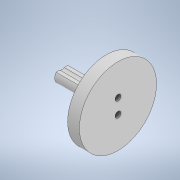
# Autodesk Inventor part: engine_gear_connector
Saved by Autodesk Inventor 2020.1 (Build 241239000, 239)
## iProperties
Created: 2022-03-03
Part Number: engine_gear_connector
Material: Generic
Document SubType Name: Modeling
Designer: OEM
Density: 1 g/cm^3
Appearance: Default
Author: OEM
Autodesk Inventor part; units mm, degrees
ref_plane "YZ Plane" through (0, 0, 0) normal (1, 0, 0) x (0, 1, 0)
ref_plane "XZ Plane" through (0, 0, 0) normal (0, 1, 0) x (-1, 0, 0)
ref_plane "XY Plane" through (0, 0, 0) normal (0, 0, 1) x (1, 0, 0)
sketch "Sketch1" plane through (0, 0, 0) normal (1, 0, 0) x (0, 1, 0)
  circle A0 centre (0, 0) radius 13.1
  circle A1 centre (0, 0) radius 2.5
  line L0 (16, 0) -> (-16, 0) construction
  circle A2 centre (-2.5, 0) radius 1
  circle A3 centre (2.5, 0) radius 1
  line L1 (1.5, 2) -> (1.5, -2)
  circle A4 centre (2.5, 0) radius 1.25
  circle A5 centre (-2.5, 0) radius 1.25
  point P0 (-2.3, 0.9798)
  point P1 (-2.3, -0.9798)
  point P2 (-2.1875, 1.2103)
  point P3 (-2.1875, -1.2103)
  point P4 (1.5, -0.75)
  point P5 (1.5, 0.75)
  dimension "d0" = 26.2
  dimension "d1" = 5
  dimension "d2" = 2
  dimension "d3" = 2
  dimension "d9" = 2.5
  dimension "d10" = 2.5
  constraints: 6 centre point, 4 coincident, 4 end point, 4 point on circle, 1 horizontal, 1 point on line, 1 vertical
  measures "d0" diameter of A0
  measures "d1" diameter of A1
  measures "d2" diameter of A2
  measures "d3" diameter of A3
  measures "d9" diameter of A4
  measures "d10" diameter of A5
extrude "Extrusion1" add sketch "Sketch1" along normal blind 4 contours A0 | A3 L1 A4 A1 | A1 A4 A3 | A1 A4 L1 A3 | A4 L1 A1 | L1 A4 | A1 L1 A4 | L1 A4 A1 A5 | A5 A1 A2 | A1 A2 A5
extrude "Extrusion3" add sketch "Sketch1" against normal blind 15 contours L1 A4 A1 A5
fillet "Fillet2" radius 1 2 edges at (0, -3.5, 0) (0, 1.5, 0)
body "Solid1"
